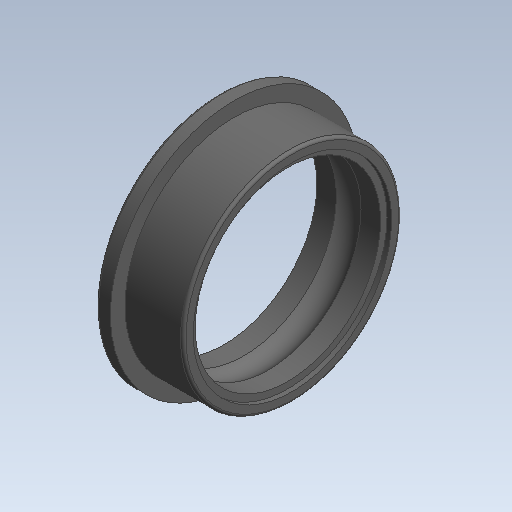
# Autodesk Inventor part: MF126ZZ Outer Ring
Saved by Autodesk Inventor 2020.2 (Build 242310000, 310)
## iProperties
Part Number: MF126ZZ Outer Ring
Material: 一般
Catalog Web Link: www.cadenas.de
Description: shielded_type_zz_zzs_OR-
Vendor: NSK_RB
Document SubType Name: Modeling
Designer: partserver
Manufacturer: NSK_RB
Mass: 0.136286 g
Surface Area: 4.13802 cm^2
Volume: 0.136286 cm^3
Density: 1 g/cm^3
Appearance: PSOLRGB-128-128-128
Category: PARTsolutions
Company: NSK_RB
PSOL_IDENT_0: {$CADENAS_DATA\23d-libs\nsk_rb\roller_bearings\deep_groove_bb\exstra_small_miniatur_bb\metric_design
PSOL_IDENT_1: _with_flange\shielded_type_zz_zzs_or1.prj},194 {VTYP=3D},{NB=MF126ZZ Outer Ring},{LINA=MF126ZZ Outer
PSOL_IDENT_2: Ring},{NN=shielded_type_zz_zzs_OR},{DATE=10.04.2020 04:57:39},{GEOMDATE=04.01.2008 00:00:00},{VERSI
PSOL_IDENT_3: ON=},{LINEID=570},{WBVAR=},{WBNUMERIC=}  {NB=MF126ZZ Outer Ring},{LINA=MF126ZZ Outer Ring},{KT=DUMMY
PSOL_IDENT_4: },{IDNR=},{STAN=},{ORDER=MF126ZZ},{SD=6.0},{X=6.0},{D=12},{DD=12},{DD1=0.0},{D2=13.6},{DD2=13.6},{B=
PSOL_IDENT_5: 0.0},{B1=4.0},{CC1=0.0},{C2=0.8},{CC2=0.8},{R=0.00},{R1=0.15},{DI1=7.73},{DI2=7.20},{SDE1=10.19},{SD
PSOL_IDENT_6: E2=10.90},{CR1=715},{COR1=292},{CR2=73},{COR2=30.0},{LG=43000},{LO=50000},{DA=0.0},{DB=7.2},{RA=0.00
PSOL_IDENT_7: },{RB=0.15},{MASS=1.94},{SC=1}
NB: MF126ZZ Outer Ring
NN: shielded_type_zz_zzs_OR
NBSYN: $ORDER. Outer Ring
LINA: MF126ZZ Outer Ring
CATALOG: NSK Rolling Bearing
ORDER: MF126ZZ
SD: 6
X: 6
D: 12
DD: 12
DD1: 0
D2: 13.6
DD2: 13.6
B: 0
B1: 4
CC1: 0
C2: 0.8
CC2: 0.8
R: 0
R1: 0.15
DI1: 7.73
DI2: 7.2
SDE1: 10.19
SDE2: 10.9
CR1: 715
COR1: 292
CR2: 73
COR2: 30
LG: 43000
LO: 50000
DA: 0
DB: 7.2
RA: 0
RB: 0.15
MASS: 1.94
SC: 1
SUPPLIER: NSK_RB
ARTICLENO: MF126ZZ Outer Ring
BOMINFO: MF126ZZ Outer Ring
CREATOR: CADENAS GmbH
Title: MF126ZZ Outer Ring
Author: Cadenas PARTsolutions
Autodesk Inventor part; units mm, degrees
sketch "Sketch_1" plane through (0, 0, 0) normal (0, 0, 1) x (1, 0, 0)
  line L0 (4, 0) -> (0, 0)
  line L1 (0, 5.45) -> (0.25, 5.45)
  line L2 (0.25, 5.45) -> (0.25, 5.095)
  line L3 (0.25, 5.095) -> (1.3247, 5.095)
  arc A0 (2.6753, 5.095) -> (1.3247, 5.095) centre (2, 4.5) ccw
  line L4 (2.6753, 5.095) -> (3.75, 5.095)
  line L5 (3.75, 5.095) -> (3.75, 5.45)
  line L6 (3.75, 5.45) -> (4, 5.45)
  line L7 (4, 5.45) -> (4, 6.65)
  arc A1 (4, 6.65) -> (3.85, 6.8) centre (3.85, 6.65) ccw
  line L8 (3.85, 6.8) -> (3.2, 6.8)
  line L9 (3.2, 6.8) -> (3.2, 6)
  line L10 (3.2, 6) -> (0.15, 6)
  arc A2 (0.15, 6) -> (0, 5.85) centre (0.15, 5.85) ccw
  line L11 (0, 5.85) -> (0, 5.45)
  constraints: 24 end point, 6 point on circle, 3 centre point
revolve "Revolution1" add sketch "Sketch_1" angle 360 about axis through (4, 0, 0) along (1, 0, 0)
ref_plane "ip_st_1_XY" through (0, 0, 0) normal (1, 0, 0) x (0, 0, -1)
ref_plane "ip_st_1_YZ" through (0, 0, 0) normal (0, 0, -1) x (0, 1, 0)
ref_plane "ip_st_1_ZX" through (0, 0, 0) normal (0, 1, 0) x (1, 0, 0)
ref_plane "ip_st_2_XY" through (3.75, 0, 0) normal (-1, 0, 0) x (0, 0, -1)
ref_plane "ip_st_2_YZ" through (3.75, 0, 0) normal (0, 0, -1) x (0, -1, 0)
ref_plane "ip_st_2_ZX" through (3.75, 0, 0) normal (0, -1, 0) x (-1, 0, 0)
body "Solid1"
